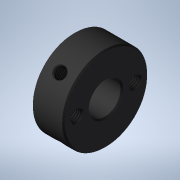
# Autodesk Inventor part: SCTW12b
Saved by Autodesk Inventor 2021 (Build 250183000, 183)
## iProperties
Created: 2025-04-29
Part Number: SCTW12b
Material: Generic
Catalog Web Link: www.cadenas.de
Description: SCTW, PSCTW, SSCTW-b-Shaft Collars - Set Screw, with 2 Holes
Vendor: MISUMI
Document SubType Name: Modeling
Designer: psAdmin
Manufacturer: MISUMI
Mass: 7.65442 g
Surface Area: 34.0596 cm^2
Volume: 7.65442 cm^3
Density: 1 g/cm^3
Appearance: PSOLRGB-175-175-175
Category: PARTsolutions
Company: MISUMI
Title: SCTW12
Author: Cadenas PARTsolutions
Comments: Shaft Collars - Set Screw, with 2 Holes
PSOL_IDENT_0: {$CADENAS_DATA/23d-libs/misumi/metric/03_set_collars/sctw/sctw_b.prj},173 {VTYP=3D},{NB=SCTW12b},{LI
PSOL_IDENT_1: NA=SCTW12},{NN=SCTW, PSCTW, SSCTW-b},{DATE=02.06.2021 03:00:04},{GEOMDATE=25.12.2015 07:47:56},{VERS
PSOL_IDENT_2: ION=},{LINEID=70},{WBVAR=MAT,ST},{WBNUMERIC=}  {NB=SCTW12b},{LINA=SCTW12},{KT=DUMMY},{PN=SCTW12},{TY
PSOL_IDENT_3: PE=SCTW},{MAT=1045},{ST=Black Oxide},{AC=Set Screws 2 Pcs.},{D=12},{B=12},{D1=32},{P=22},{M=M5x5},{T
PSOL_IDENT_4: HMD=5},{THDMIN=4.134},{M1=M5},{M1NDM=5},{C=0.5},{ST0='Black Oxide','Black Oxide','Electroless Nickel
PSOL_IDENT_5: Plating','Electroless Nickel Plating'},{L=5}
NB: SCTW12b
NN: SCTW, PSCTW, SSCTW-b
NT: Shaft Collars - Set Screw, with 2 Holes
NBSYN: $PN.b
LINA: SCTW12
CATALOG: Misumi
PN: SCTW12
MAT: S45C Equivalent
ST: Black Oxide
AC: Set Screws 2 Pcs.
D: 12
B: 12
D1: 32
P: 22
M: M5x5
M1: M5
SUPPLIER: MISUMI
ARTICLENO: SCTW12b
BOMINFO: SCTW12
CREATOR: CADENAS GmbH
Autodesk Inventor part; units mm, degrees
sketch "Sketch_1" plane through (0, 0, 0) normal (0, 0, 1) x (1, 0, 0)
  line L0 (0, 0) -> (-6, 0)
  line L1 (-6, 6.5) -> (-5.5, 6)
  line L2 (-5.5, 6) -> (5.5, 6)
  line L3 (5.5, 6) -> (6, 6.5)
  line L4 (6, 6.5) -> (6, 15.5)
  line L5 (6, 15.5) -> (5.5, 16)
  line L6 (5.5, 16) -> (-5.5, 16)
  line L7 (-5.5, 16) -> (-6, 15.5)
  line L8 (-6, 15.5) -> (-6, 6.5)
  constraints: 18 end point
revolve "Revolution1" add sketch "Sketch_1" angle 360 about axis through (0, 0, 0) along (1, 0, 0)
sketch "Sketch_2" plane through (0, 0, 0) normal (1, 0, 0) x (0, 1, 0)
  line L0 (12.4451, 12.4451) -> (3.1113, 3.1113)
  line L1 (3.1113, 3.1113) -> (1.3435, 4.879)
  line L2 (1.3435, 4.879) -> (2.4749, 6.0104)
  line L3 (2.4749, 6.0104) -> (3.0872, 6.0104)
  line L4 (3.0872, 6.0104) -> (9.5459, 12.4691)
  line L5 (9.5459, 12.4691) -> (9.5459, 13.0815)
  line L6 (9.5459, 13.0815) -> (10.6773, 14.2128)
  line L7 (10.6773, 14.2128) -> (12.4451, 12.4451)
  line L8 (12.4451, 12.4451) -> (3.1113, 3.1113)
  constraints: 18 end point
revolve "Revolution2" cut sketch "Sketch_2" angle 360 about axis through (0, 12.4451, 12.4451) along (0, 0.7071068, 0.7071068)
thread "Thread1" size "M5x0.8" class "6H" standard "ISO Metric profile" full length
sketch "Sketch_3" plane through (0, 0, 0) normal (1, 0, 0) x (0, 1, 0)
  line L0 (-12.4451, 12.4451) -> (-3.1113, 3.1113)
  line L1 (-3.1113, 3.1113) -> (-4.879, 1.3435)
  line L2 (-4.879, 1.3435) -> (-6.0104, 2.4749)
  line L3 (-6.0104, 2.4749) -> (-6.0104, 3.0872)
  line L4 (-6.0104, 3.0872) -> (-12.4691, 9.5459)
  line L5 (-12.4691, 9.5459) -> (-13.0815, 9.5459)
  line L6 (-13.0815, 9.5459) -> (-14.2128, 10.6773)
  line L7 (-14.2128, 10.6773) -> (-12.4451, 12.4451)
  line L8 (-12.4451, 12.4451) -> (-3.1113, 3.1113)
  constraints: 18 end point
revolve "Revolution3" cut sketch "Sketch_3" angle 360 about axis through (0, -12.4451, 12.4451) along (0, -0.7071068, 0.7071068)
thread "Thread2" size "M5x0.8" class "6H" standard "ISO Metric profile" full length
sketch "Sketch_5" plane through (0, 0, 0) normal (0, 1, 0) x (-1, 0, 0)
  line L0 (-6, -11) -> (6, -11)
  line L1 (6, -11) -> (6, -13.5)
  line L2 (6, -13.5) -> (5.567, -13.067)
  line L3 (5.567, -13.067) -> (-5.567, -13.067)
  line L4 (-5.567, -13.067) -> (-6, -13.5)
  line L5 (-6, -13.5) -> (-6, -11)
  line L6 (-6, -11) -> (6, -11)
  constraints: 14 end point
revolve "Revolution4" cut sketch "Sketch_5" angle 360 about axis through (6, 0, -11) along (1, 0, 0)
thread "Thread3" size "M5x0.8" class "6H" standard "ISO Metric profile" full length
sketch "Sketch_9" plane through (0, 0, 0) normal (0, 1, 0) x (-1, 0, 0)
  line L0 (-6, 11) -> (6, 11)
  line L1 (6, 11) -> (6, 8.5)
  line L2 (6, 8.5) -> (5.567, 8.933)
  line L3 (5.567, 8.933) -> (-5.567, 8.933)
  line L4 (-5.567, 8.933) -> (-6, 8.5)
  line L5 (-6, 8.5) -> (-6, 11)
  line L6 (-6, 11) -> (6, 11)
  constraints: 14 end point
revolve "Revolution5" cut sketch "Sketch_9" angle 360 about axis through (6, 0, 11) along (1, 0, 0)
thread "Thread4" size "M5x0.8" class "6H" standard "ISO Metric profile" full length
ref_plane "body_set_h_XY" through (0, -11.3137, 11.3137) normal (0, 0.7071068, -0.7071068) x (1, 0, 0)
ref_plane "body_set_h_YZ" through (0, -11.3137, 11.3137) normal (1, 0, 0) x (0, -0.7071068, -0.7071068)
ref_plane "body_set_h_ZX" through (0, -11.3137, 11.3137) normal (0, -0.7071068, -0.7071068) x (0, 0.7071068, -0.7071068)
ref_plane "body_set_v_XY" through (0, 11.3137, 11.3137) normal (0, 0.7071068, 0.7071068) x (1, 0, 0)
ref_plane "body_set_v_YZ" through (0, 11.3137, 11.3137) normal (1, 0, 0) x (0, 0.7071068, -0.7071068)
ref_plane "body_set_v_ZX" through (0, 11.3137, 11.3137) normal (0, 0.7071068, -0.7071068) x (0, 0.7071068, 0.7071068)
body "Solid1"
